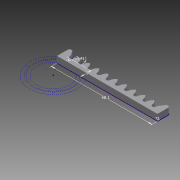
# Autodesk Inventor part: TestRack
Saved by Autodesk Inventor 2014 SP1 (Build 180222100, 222)
## iProperties
Created: 2014-06-08
Part Number: TestRack
Material: Generic
Document SubType Name: Modeling
Designer: Erin
Density: 1 g/cm^3
Appearance: Default
Author: Erin
Autodesk Inventor part; units mm, degrees
ref_plane "YZ Plane" through (0, 0, 0) normal (1, 0, 0) x (0, 1, 0)
ref_plane "XZ Plane" through (0, 0, 0) normal (0, 1, 0) x (-1, 0, 0)
ref_plane "XY Plane" through (0, 0, 0) normal (0, 0, 1) x (1, 0, 0)
sketch "Sketch1" plane through (0, 0, 0) normal (0, 0, 1) x (1, 0, 0)
  spline S0 degree 3 poles (-2.2049, 11.0052) (-2.1366, 10.9392) (-1.9999, 10.8072) (-1.8073, 10.5969) (-1.6248, 10.3779) (-1.4549, 10.149) (-1.2994, 9.91) (-1.1842, 9.702) (-1.103, 9.5302) (-1.0489, 9.3984) (-1.0013, 9.2639) (-0.9809, 9.171) (-0.9707, 9.1246) knots 0 0 0 0 0.028496 0.056993 0.085489 0.113985 0.142479 0.170971 0.18522 0.199468 0.213715 0.227956 0.227956 0.227956 0.227956
  spline S1 degree 3 poles (-0.9707, 9.1246) (-0.9683, 9.0496) (-0.9649, 8.9371) (-0.9464, 8.7881) (-0.9248, 8.6776) (-0.8975, 8.5684) (-0.8609, 8.4619) (-0.8165, 8.3583) (-0.7616, 8.2599) (-0.6963, 8.168) (-0.6206, 8.0845) (-0.5344, 8.0117) (-0.4384, 7.9523) (-0.3345, 7.9083) (-0.225, 7.8806) (-0.1124, 7.873) (0, 7.876) (0.1124, 7.873) (0.225, 7.8806) (0.3345, 7.9083) (0.4384, 7.9523) (0.5344, 8.0117) (0.6206, 8.0845) (0.6963, 8.168) (0.7616, 8.2599) (0.8165, 8.3583) (0.8609, 8.4619) (0.8975, 8.5684) (0.9248, 8.6776) (0.9464, 8.7881) (0.9649, 8.9371) (0.9683, 9.0496) (0.9707, 9.1246) knots 0 0 0 0 0.022498 0.03375 0.045 0.056252 0.067501 0.078751 0.090002 0.10125 0.112496 0.12374 0.134984 0.146226 0.157462 0.168701 0.179952 0.191204 0.202442 0.213679 0.22492 0.236164 0.247408 0.258654 0.269902 0.281153 0.292403 0.303652 0.314904 0.326155 0.337406 0.359904 0.359904 0.359904 0.359904
  spline S2 degree 3 poles (0.9707, 9.1246) (0.9809, 9.171) (1.0013, 9.2639) (1.0489, 9.3984) (1.103, 9.5302) (1.1842, 9.702) (1.2994, 9.91) (1.4549, 10.149) (1.6248, 10.3779) (1.8073, 10.5969) (1.9999, 10.8072) (2.1366, 10.9392) (2.2049, 11.0052) knots 0 0 0 0 0.014241 0.028488 0.042736 0.056984 0.085476 0.113971 0.142466 0.170963 0.199459 0.227956 0.227956 0.227956 0.227956
  circle A0 centre (0, 0) radius 7.875 construction
  circle A1 centre (0, 0) radius 9.162 construction
  circle A2 centre (0, 0) radius 9.75 construction
  circle A3 centre (0, 0) radius 11.2239 construction
  line L0 (-4.2049, 11.0052) -> (-2.2049, 11.0052)
  line L1 (-4.2049, 6.0052) -> (43.8951, 6.0052)
  line L2 (-4.2049, 6.0052) -> (-4.2049, 11.0052)
  line L3 (43.8951, 6.0052) -> (43.8951, 11.0052)
  arc A4 (-2.2049, 11.0052) -> (-4.2049, 11.0052) centre (-3.2049, 11.0052) ccw
  line L4 (41.8951, 11.0052) -> (41.8951, 6.0052) construction
  arc A5 (43.8951, 11.0052) -> (41.8951, 11.0052) centre (42.8951, 11.0052) ccw
  line L5 (2.2049, 11.0052) -> (43.8951, 11.0052)
  line L6 (-2.2049, 11.0052) -> (2.2049, 11.0052)
  point P0 (-2.002, 10.8051)
  point P1 (-1.809, 10.5955)
  point P2 (-1.6269, 10.3763)
  point P3 (-1.4573, 10.1473)
  point P4 (-1.3022, 9.9082)
  point P5 (-1.1648, 9.6586)
  point P6 (-1.1041, 9.5297)
  point P7 (-1.05, 9.3979)
  point P8 (-1.0041, 9.2631)
  point P9 (-0.9591, 8.8999)
  point P10 (-0.9451, 8.7883)
  point P11 (-0.9239, 8.6778)
  point P12 (-0.896, 8.5688)
  point P13 (-0.8596, 8.4624)
  point P14 (-0.8148, 8.3592)
  point P15 (-0.7599, 8.261)
  point P16 (-0.6946, 8.1694)
  point P17 (-0.6189, 8.0862)
  point P18 (-0.5328, 8.0139)
  point P19 (-0.4371, 7.9548)
  point P20 (-0.3336, 7.911)
  point P21 (-0.2245, 7.884)
  point P22 (-0.1125, 7.8748)
  point P23 (0, 7.875)
  point P24 (0.1125, 7.8748)
  point P25 (0.2245, 7.884)
  point P26 (0.3336, 7.911)
  point P27 (0.4371, 7.9548)
  point P28 (0.5328, 8.0139)
  point P29 (0.6189, 8.0862)
  point P30 (0.6946, 8.1694)
  point P31 (0.7599, 8.261)
  point P32 (0.8148, 8.3592)
  point P33 (0.8596, 8.4624)
  point P34 (0.896, 8.5688)
  point P35 (0.9239, 8.6778)
  point P36 (0.9451, 8.7883)
  point P37 (0.9591, 8.8999)
  point P38 (1.0041, 9.2631)
  point P39 (1.05, 9.3979)
  point P40 (1.1041, 9.5297)
  point P41 (1.1648, 9.6586)
  point P42 (1.3022, 9.9082)
  point P43 (1.4573, 10.1473)
  point P44 (1.6269, 10.3763)
  point P45 (1.809, 10.5955)
  point P46 (2.002, 10.8051)
  dimension "d2" = 5
  dimension "d3" = 48.1
  dimension "d4" = 2
  dimension "d5" = 4.4097
  dimension "d6" = 2
  constraints: 14 end point, 6 centre point, 6 horizontal, 6 point on circle, 3 point on line, 3 tangent, 2 perpendicular, 1 parallel, 110 other
  measures "d2" distance between parallel lines of L1 L0
  measures "d3" distance of L1.start L1.end
  measures "d4" distance from line of L0.end L2
  measures "d5" distance of L5.start L0.end
  measures "d6" distance between parallel lines of L4 L3
extrude "Extrusion2" add sketch "Sketch1" along normal blind 3
extrude "Extrusion3" cut sketch "Sketch1" along normal blind 3 contours L6 S2 S1 S0
pattern_linear "Rectangular Pattern1" count 10 spacing 4.41 along (1, 0, 0) of "Extrusion3"
equation "\"Module\" = 1.5"
equation "\"PressureAngle\" = 20deg"
equation "\"UnitProfileClearance\" = 0.25"
equation "\"UnitRoundRadius\" = 0.35"
equation "\"HeadDiameter\" = 22.44787"
equation "\"RootDiameter\" = 15.75"
equation "\"BaseDiameter\" = 18.32401"
equation "\"PitchDiameter\" = 19.5"
equation "\"FaceWidth\" = 3"
equation "\"HelixAngle\" = 0"
equation "\"UnitCorrection\" = 0"
equation "\"UnitAddendumModification\" = 0.017376"
equation "\"CircularPitch\" = 4.712389"
equation "\"UnitBacklashShift\" = 0"
equation "\"TotalToolShift\" = 0"
equation "\"IsInternal\" = 0"
body "Solid2"
